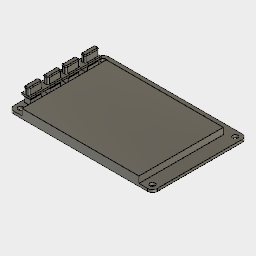
2423 PiTFT 2.8 (Autodesk Fusion 360 design; units mm, degrees)
Autodesk Fusion 360 part; units mm, degrees
note: some values were not read from the file. Chosen so that the rebuilt part matches the saved one: which face or edge a step refers to.
sketch "pcb" plane through (0, 0, 0) normal (0, 0, 1) x (1, 0, 0)
  line L0 (0, 0) -> (85, 0)
  line L1 (85, 0) -> (85, -56)
  line L2 (85, -56) -> (0, -56)
  line L3 (0, -56) -> (0, 0)
  circle A0 centre (3.5, -3.5) radius 1.5
  line L4 (42.5, 0) -> (42.5, -56) construction
  line L5 (85, -28) -> (0, -28) construction
  circle A1 centre (81.5, -3.5) radius 1.5
  circle A2 centre (3.5, -52.5) radius 1.5
  circle A3 centre (81.5, -52.5) radius 1.5
  line L6 (7.8, -6.1) -> (77, -6.1)
  line L7 (77, -6.1) -> (77, -56)
  line L8 (77, -56) -> (7.8, -56)
  line L9 (7.8, -56) -> (7.8, -6.1)
  line L10 (10.2, -8.5) -> (69.7, -8.5)
  line L11 (69.7, -8.5) -> (69.7, -53.5)
  line L12 (69.7, -53.5) -> (10.2, -53.5)
  line L13 (10.2, -53.5) -> (10.2, -8.5)
  line L14 (5.25, -48.3) -> (1.75, -48.3)
  line L15 (1.75, -48.3) -> (1.75, -42.1)
  line L16 (1.75, -42.1) -> (5.25, -42.1)
  line L17 (5.25, -42.1) -> (5.25, -48.3)
  line L18 (5.25, -48.3) -> (1.75, -42.1) construction
  line L19 (1.75, -48.3) -> (5.25, -42.1) construction
  line L20 (5.25, -36.87) -> (1.75, -36.87)
  line L21 (1.75, -36.87) -> (1.75, -30.67)
  line L22 (1.75, -30.67) -> (5.25, -30.67)
  line L23 (5.25, -30.67) -> (5.25, -36.87)
  line L24 (5.25, -36.87) -> (1.75, -30.67) construction
  line L25 (1.75, -36.87) -> (5.25, -30.67) construction
  line L26 (5.25, -26.08) -> (1.75, -26.08)
  line L27 (1.75, -26.08) -> (1.75, -19.88)
  line L28 (1.75, -19.88) -> (5.25, -19.88)
  line L29 (5.25, -19.88) -> (5.25, -26.08)
  line L30 (5.25, -26.08) -> (1.75, -19.88) construction
  line L31 (1.75, -26.08) -> (5.25, -19.88) construction
  line L32 (5.25, -14.65) -> (1.75, -14.65)
  line L33 (1.75, -14.65) -> (1.75, -8.45)
  line L34 (1.75, -8.45) -> (5.25, -8.45)
  line L35 (5.25, -8.45) -> (5.25, -14.65)
  line L36 (5.25, -14.65) -> (1.75, -8.45) construction
  line L37 (1.75, -14.65) -> (5.25, -8.45) construction
  circle A4 centre (61.5, -3.5) radius 1.5
  line L38 (57.8, -5.8) -> (7.2, -5.8)
  line L39 (7.2, -5.8) -> (7.2, -0.8)
  line L40 (7.2, -0.8) -> (57.8, -0.8)
  line L41 (57.8, -0.8) -> (57.8, -5.8)
  line L42 (57.8, -5.8) -> (7.2, -0.8) construction
  line L43 (7.2, -5.8) -> (57.8, -0.8) construction
  point P0 (3.5, -45.2)
  point P1 (3.5, -33.77)
  point P2 (3.5, -22.98)
  point P3 (3.5, -11.55)
  point P4 (32.5, -3.3)
  dimension "d1" = 85
  dimension "d2" = 56
  dimension "d3" = 3
  dimension "d4" = 3.5
  dimension "d5" = 3.5
  dimension "d6" = 69.2
  dimension "d7" = 49.9
  dimension "d8" = 7.8
  dimension "d9" = 45
  dimension "d10" = 59.5
  dimension "d11" = 2.4
  dimension "d12" = 2.4
  dimension "d13" = 6.2
  dimension "d14" = 3.5
  dimension "d15" = 3.5
  dimension "d16" = 10.8
  dimension "d17" = 6.2
  dimension "d18" = 3.5
  dimension "d20" = 22.23
  dimension "d21" = 6.2
  dimension "d22" = 3.5
  dimension "d23" = 33.02
  dimension "d24" = 3.5
  dimension "d25" = 6.2
  dimension "d26" = 44.45
  dimension "d34" = 3
  dimension "d35" = 58
  dimension "d92" = 50.6
  dimension "d93" = 5
  dimension "d94" = 0.8
  dimension "d95" = 7.2
  measures "d1" distance of L0.start L0.end
  measures "d2" distance of L0.start L2.end
  measures "d3" diameter of A0
  measures "d4" distance of L3 A0.centre
  measures "d5" distance of L0 A0.centre
  measures "d6" distance of L6.start L6.end
  measures "d7" distance of L6.start L8.end
  measures "d8" distance of L3 L9
  measures "d9" distance of L10.start L12.end
  measures "d10" distance of L10.start L10.end
  measures "d11" distance of L6 L10
  measures "d12" distance of L9 L13
  measures "d13" distance of L14.end L15.end
  measures "d14" distance of L15.end L16.end
  measures "d15" distance of L3 P0
  measures "d16" distance of L2 P0
  measures "d17" distance of L20.end L21.end
  measures "d18" distance of L21.end L22.end
  measures "d20" distance of L2 P1
  measures "d21" distance of L26.end L27.end
  measures "d22" distance of L27.end L28.end
  measures "d23" distance of L2 P2
  measures "d24" distance of L33.end L34.end
  measures "d25" distance of L32.end L33.end
  measures "d26" distance of L2 P3
  measures "d34" diameter of A4
  measures "d35" distance of A0.centre A4.centre
  measures "d92" distance of L39.end L40.end
  measures "d93" distance of L38.end L39.end
  measures "d94" distance of L0 L40
  measures "d95" distance of L3 L39
extrude "Extrude1" add sketch "pcb" against normal blind 1.6 contours L0 L1 L2 L3 L6 L7 L9 | L2 L6 L7 L8 L9 | L10 L11 L12 L13 | L14 L15 L16 L17 | L20 L21 L22 L23 | L26 L27 L28 L29 | L32 L33 L34 L35 | L38 L39 L40 L41 makes body 1
extrude "Extrude2" add sketch "pcb" along normal blind 3.8 contours L2 L6 L7 L8 L9 | L10 L11 L12 L13 bodies 1
extrude "Extrude3" add sketch "pcb" along normal blind 3 contours L14 L15 L16 L17 | L20 L21 L22 L23 | L26 L27 L28 L29 | L32 L33 L34 L35 bodies 1
fillet "Fillet1" radius 3 4 edges at (0, 0, -0.8) (0, -56, -0.8) (85, -56, -0.8) (85, 0, -0.8) on bodies 1
sketch "mount" plane through (0, 0, 0) normal (0, 0, 1) x (1, 0, 0)
  line L0 (0, 0) -> (85, 0)
  line L1 (85, 0) -> (85, -56)
  line L2 (85, -56) -> (0, -56)
  line L3 (0, -56) -> (0, 0)
  circle A0 centre (3.5, -3.5) radius 1.4
  circle A1 centre (61.5, -3.5) radius 1.5
  line L4 (42.5, 0) -> (42.5, -56) construction
  line L5 (0, -28) -> (85, -28) construction
  circle A2 centre (81.5, -3.5) radius 1.4
  circle A3 centre (3.5, -52.5) radius 1.4
  circle A4 centre (81.5, -52.5) radius 1.4
  line L6 (87, -58) -> (-2, -58)
  line L7 (-2, -58) -> (-2, 2)
  line L8 (-2, 2) -> (87, 2)
  line L9 (87, 2) -> (87, -58)
  line L10 (1, -6) -> (6, -6)
  line L11 (6, -6) -> (6, -50.5)
  line L12 (6, -50.5) -> (1, -50.5)
  line L13 (1, -50.5) -> (1, -6)
  dimension "d36" = 85
  dimension "d37" = 56
  dimension "d38" = 2.8
  dimension "d39" = 3.5
  dimension "d40" = 3.5
  dimension "d41" = 3
  dimension "d42" = 58
  dimension "d43" = 5
  dimension "d44" = 44.5
  measures "d36" distance of L0.start L0.end
  measures "d37" distance of L0.start L2.end
  measures "d38" diameter of A0
  measures "d39" distance of L3 A0.centre
  measures "d40" distance of L0 A0.centre
  measures "d41" diameter of A1
  measures "d42" distance of A0.centre A1.centre
  measures "d43" distance of L10.start L10.end
  measures "d44" distance of L10.start L12.end
sketch "buttons" plane through (0, 0, 0) normal (0, 0, 1) x (1, 0, 0)
  line L0 (4, -16.3) -> (3, -16.3)
  line L1 (1.5, -14.8) -> (1.5, -8.3)
  line L2 (3, -6.8) -> (4, -6.8)
  line L3 (5.5, -8.3) -> (5.5, -14.8)
  line L4 (5.5, -16.3) -> (1.5, -6.8) construction
  line L5 (1.5, -16.3) -> (5.5, -6.8) construction
  line L6 (4, -27.73) -> (3, -27.73)
  line L7 (1.5, -26.23) -> (1.5, -19.73)
  line L8 (3, -18.23) -> (4, -18.23)
  line L9 (5.5, -19.73) -> (5.5, -26.23)
  line L10 (5.5, -27.73) -> (1.5, -18.23) construction
  line L11 (1.5, -27.73) -> (5.5, -18.23) construction
  line L12 (4, -38.52) -> (3, -38.52)
  line L13 (1.5, -37.02) -> (1.5, -30.52)
  line L14 (3, -29.02) -> (4, -29.02)
  line L15 (5.5, -30.52) -> (5.5, -37.02)
  line L16 (5.5, -38.52) -> (1.5, -29.02) construction
  line L17 (1.5, -38.52) -> (5.5, -29.02) construction
  line L18 (4, -49.95) -> (3, -49.95)
  line L19 (1.5, -48.45) -> (1.5, -41.95)
  line L20 (3, -40.45) -> (4, -40.45)
  line L21 (5.5, -41.95) -> (5.5, -48.45)
  line L22 (5.5, -49.95) -> (1.5, -40.45) construction
  line L23 (1.5, -49.95) -> (5.5, -40.45) construction
  arc A0 (3, -6.8) -> (1.5, -8.3) centre (3, -8.3) ccw
  arc A1 (5.5, -8.3) -> (4, -6.8) centre (4, -8.3) ccw
  arc A2 (4, -16.3) -> (5.5, -14.8) centre (4, -14.8) ccw
  arc A3 (1.5, -14.8) -> (3, -16.3) centre (3, -14.8) ccw
  arc A4 (3, -18.23) -> (1.5, -19.73) centre (3, -19.73) ccw
  arc A5 (5.5, -19.73) -> (4, -18.23) centre (4, -19.73) ccw
  arc A6 (4, -27.73) -> (5.5, -26.23) centre (4, -26.23) ccw
  arc A7 (1.5, -26.23) -> (3, -27.73) centre (3, -26.23) ccw
  arc A8 (5.5, -30.52) -> (4, -29.02) centre (4, -30.52) ccw
  arc A9 (3, -29.02) -> (1.5, -30.52) centre (3, -30.52) ccw
  arc A10 (1.5, -37.02) -> (3, -38.52) centre (3, -37.02) ccw
  arc A11 (4, -38.52) -> (5.5, -37.02) centre (4, -37.02) ccw
  arc A12 (3, -40.45) -> (1.5, -41.95) centre (3, -41.95) ccw
  arc A13 (5.5, -41.95) -> (4, -40.45) centre (4, -41.95) ccw
  arc A14 (4, -49.95) -> (5.5, -48.45) centre (4, -48.45) ccw
  arc A15 (1.5, -48.45) -> (3, -49.95) centre (3, -48.45) ccw
  arc A16 (5, -8.3) -> (4, -7.3) centre (4, -8.3) ccw
  line L24 (3, -7.3) -> (4, -7.3)
  arc A17 (3, -7.3) -> (2, -8.3) centre (3, -8.3) ccw
  line L25 (2, -14.8) -> (2, -8.3)
  arc A18 (2, -14.8) -> (3, -15.8) centre (3, -14.8) ccw
  line L26 (4, -15.8) -> (3, -15.8)
  arc A19 (4, -15.8) -> (5, -14.8) centre (4, -14.8) ccw
  line L27 (5, -8.3) -> (5, -14.8)
  line L28 (3, -18.73) -> (4, -18.73)
  arc A20 (5, -19.73) -> (4, -18.73) centre (4, -19.73) ccw
  line L29 (5, -19.73) -> (5, -26.23)
  arc A21 (4, -27.23) -> (5, -26.23) centre (4, -26.23) ccw
  line L30 (4, -27.23) -> (3, -27.23)
  arc A22 (2, -26.23) -> (3, -27.23) centre (3, -26.23) ccw
  line L31 (2, -26.23) -> (2, -19.73)
  arc A23 (3, -18.73) -> (2, -19.73) centre (3, -19.73) ccw
  arc A24 (5, -30.52) -> (4, -29.52) centre (4, -30.52) ccw
  line L32 (3, -29.52) -> (4, -29.52)
  arc A25 (3, -29.52) -> (2, -30.52) centre (3, -30.52) ccw
  line L33 (2, -37.02) -> (2, -30.52)
  arc A26 (2, -37.02) -> (3, -38.02) centre (3, -37.02) ccw
  line L34 (4, -38.02) -> (3, -38.02)
  arc A27 (4, -38.02) -> (5, -37.02) centre (4, -37.02) ccw
  line L35 (5, -30.52) -> (5, -37.02)
  arc A28 (5, -41.95) -> (4, -40.95) centre (4, -41.95) ccw
  line L36 (3, -40.95) -> (4, -40.95)
  arc A29 (3, -40.95) -> (2, -41.95) centre (3, -41.95) ccw
  line L37 (2, -48.45) -> (2, -41.95)
  arc A30 (2, -48.45) -> (3, -49.45) centre (3, -48.45) ccw
  line L38 (4, -49.45) -> (3, -49.45)
  arc A31 (4, -49.45) -> (5, -48.45) centre (4, -48.45) ccw
  line L39 (5, -41.95) -> (5, -48.45)
  point P0 (3.5, -11.55)
  point P1 (3.5, -11.55)
  point P2 (3.5, -22.98)
  point P3 (3.5, -22.98)
  point P4 (3.5, -33.77)
  point P5 (3.5, -33.77)
  point P6 (3.5, -45.2)
  point P7 (3.5, -45.2)
  dimension "d45" = 9.5
  dimension "d46" = 4
  dimension "d47" = 4
  dimension "d48" = 9.5
  dimension "d49" = 4
  dimension "d50" = 9.5
  dimension "d51" = 9.5
  dimension "d52" = 4
  dimension "d53" = 1.5
  dimension "d54" = 1.5
  dimension "d55" = 1.5
  dimension "d56" = 1.5
  dimension "d57" = 1.5
  dimension "d58" = 1.5
  dimension "d59" = 1.5
  dimension "d60" = 1.5
  dimension "d61" = 1.5
  dimension "d62" = 1.5
  dimension "d63" = 1.5
  dimension "d64" = 1.5
  dimension "d65" = 1.5
  dimension "d66" = 1.5
  dimension "d67" = 1.5
  dimension "d68" = 1.5
  measures "d45" distance of L5.start L4.end
  measures "d46" distance of L4.end L5.end
  measures "d47" distance of L10.end L11.end
  measures "d48" distance of L11.start L10.end
  measures "d49" distance of L16.end L17.end
  measures "d50" distance of L17.start L16.end
  measures "d51" distance of L23.start L22.end
  measures "d52" distance of L22.end L23.end
  measures "d53" radius of A0
  measures "d54" radius of A1
  measures "d55" radius of A2
  measures "d56" radius of A3
  measures "d57" radius of A4
  measures "d58" radius of A5
  measures "d59" radius of A6
  measures "d60" radius of A7
  measures "d61" radius of A8
  measures "d62" radius of A9
  measures "d63" radius of A10
  measures "d64" radius of A11
  measures "d65" radius of A12
  measures "d66" radius of A13
  measures "d67" radius of A14
  measures "d68" radius of A15
extrude "Extrude4" add sketch "mount" along normal blind 1.5 separate body contours L0 L1 L2 L3 | A0 | A1 | A2 | A3 | A4 | L6 L7 L8 L9 | L10 L11 L12 L13 makes body 2
extrude "Extrude5" cut sketch "buttons" along normal up to surface (1.5 mm away) contours L0 L1 L2 L3 A0 A1 A2 A3 | L6 L7 L8 L9 A4 A5 A6 A7 | L12 L13 L14 L15 A8 A9 A10 A11 | L18 L19 L20 L21 A12 A13 A14 A15 | A16 L24 A17 L25 A18 L26 A19 L27 | L28 A20 L29 A21 L30 A22 L31 A23 | A24 L32 A25 L33 A26 L34 A27 L35 | A28 L36 A29 L37 A30 L38 A31 L39 bodies 2
extrude "Extrude6" cut sketch "pcb" along normal up to surface (1.5 mm away) contours L10 L11 L12 L13 bodies 2
fillet "Fillet2" radius 2 8 edges at (-2, -58, 0.75) (10.2, -53.5, 0.75) (10.2, -8.5, 0.75) (-2, 2, 0.75) (87, -58, 0.75) (69.7, -53.5, 0.75) (69.7, -8.5, 0.75) (87, 2, 0.75) on bodies 2
move_body "MoveBody1" bodies 2 to x (1, 0, 0) y (0, 1, 0) z (0, 0, 1) at (0, 0, 3.8)
extrude "Extrude8" add sketch "mount" along normal blind 1 separate body contours L10 L11 L12 L13 makes body 3
extrude "Extrude9" add sketch "buttons" along normal blind 5 contours A16 L24 A17 L25 A18 L26 A19 L27 | L28 A20 L29 A21 L30 A22 L31 A23 | A24 L32 A25 L33 A26 L34 A27 L35 | A28 L36 A29 L37 A30 L38 A31 L39 bodies 3
fillet "Fillet3" radius 0.5 32 edges at (4.7071, -15.5071, 5) (5, -11.55, 5) (4.7071, -7.5929, 5) (3.5, -7.3, 5) (2.2929, -7.5929, 5) (2, -11.55, 5) (2.2929, -15.5071, 5) (3.5, -15.8, 5) (3.5, -27.23, 5) (4.7071, -26.9371, 5) (5, -22.98, 5) (4.7071, -19.0229, 5) (3.5, -18.73, 5) (2.2929, -19.0229, 5) (2, -22.98, 5) (2.2929, -26.9371, 5) (3.5, -38.02, 5) (4.7071, -37.7271, 5) (5, -33.77, 5) (4.7071, -29.8129, 5) (3.5, -29.52, 5) (2.2929, -29.8129, 5) (2, -33.77, 5) (2.2929, -37.7271, 5) (3.5, -49.45, 5) (4.7071, -49.1571, 5) (5, -45.2, 5) (4.7071, -41.2429, 5) (3.5, -40.95, 5) (2.2929, -41.2429, 5) (2, -45.2, 5) (2.2929, -49.1571, 5) on bodies 3
move_body "MoveBody3" bodies 2 to x (1, 0, 0) y (0, 1, 0) z (0, 0, 1) at (0, 0, 1.5)
move_body "MoveBody2" bodies 3 to x (1, 0, 0) y (0, 1, 0) z (0, 0, 1) at (0, 0, 4.3)
sketch "screen holder" plane through (0, 0, 0) normal (0, 0, 1) x (1, 0, 0)
  line L0 (7.8, -6.1) -> (77, -6.1)
  line L1 (77, -6.1) -> (77, -56)
  line L2 (77, -56) -> (7.8, -56)
  line L3 (7.8, -56) -> (7.8, -6.1)
  line L4 (78.5, -57.5) -> (6.3, -57.5)
  line L5 (6.3, -57.5) -> (6.3, -4.6)
  line L6 (6.3, -4.6) -> (78.5, -4.6)
  line L7 (78.5, -4.6) -> (78.5, -57.5)
  line L8 (77.2, -56.2) -> (7.6, -56.2)
  line L9 (7.6, -56.2) -> (7.6, -5.9)
  line L10 (7.6, -5.9) -> (77.2, -5.9)
  line L11 (77.2, -5.9) -> (77.2, -56.2)
  line L12 (77.4, -56.4) -> (7.4, -56.4)
  line L13 (7.4, -56.4) -> (7.4, -5.7)
  line L14 (7.4, -5.7) -> (77.4, -5.7)
  line L15 (77.4, -5.7) -> (77.4, -56.4)
  point P0 (7.8, -6.1)
  point P1 (77, -56)
extrude "Extrude10" add sketch "screen holder" along normal blind 5.3 and the other way blind -1 contours L4 L5 L6 L7 | L8 L9 L10 L11 | L12 L13 L14 L15 bodies 2
extrude "Extrude11" cut sketch "screen holder" along normal up to surface (5.3 mm away) contours L0 L1 L2 L3 | L8 L9 L10 L11 bodies 2
extrude "Extrude12" add sketch "mount" along normal blind 5.3 and the other way blind 1.6 contours A0 | A2 | A3 | A4 bodies 2
move_face "OffsetFaces1" offset 1.5 1 faces at (74.7, -37.8667, 5.3) on bodies 2
chamfer "Chamfer1" distance 1.5 angle 45 8 edges at (39.95, -8.5, 6.8) (10.7858, -9.0858, 6.8) (10.2, -31, 6.8) (10.7858, -52.9142, 6.8) (39.95, -53.5, 6.8) (69.1142, -52.9142, 6.8) (69.7, -31, 6.8) (69.1142, -9.0858, 6.8) on bodies 2
extrude "Extrude13" add sketch "pcb" against normal blind 15 contours L38 L39 L40 L41 bodies 1
move_face "OffsetFaces2" offset -1.05 1 faces at (4.3333, -50.5, 4.6333) on bodies 3
move_face "OffsetFaces3" offset -1.3 1 faces at (2.6667, -6, 4.6333) on bodies 3
hidden bodies 2
named bodies: "screen pcb", "mount", "pitft buttons"
